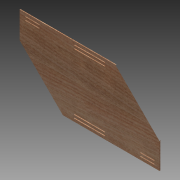
# Autodesk Inventor part: plaat
Saved by Autodesk Inventor 2015 (Build 190159000, 159)
## iProperties
Created: 2015-12-19
Part Number: plaat
Material: Generic
Document SubType Name: Modeling
Designer: david
Density: 1 g/cm^3
Appearance: Birch - Natural Polished
Author: david
Autodesk Inventor part; units mm, degrees
ref_plane "YZ Plane" through (0, 0, 0) normal (1, 0, 0) x (0, 1, 0)
ref_plane "XZ Plane" through (0, 0, 0) normal (0, 1, 0) x (-1, 0, 0)
ref_plane "XY Plane" through (0, 0, 0) normal (0, 0, 1) x (1, 0, 0)
sketch "Sketch1" plane through (0, 0, 0) normal (0, 1, 0) x (-1, 0, 0)
  line L0 (-250, 125) -> (250, 125)
  line L1 (250, 125) -> (250, -125)
  line L2 (250, -125) -> (-250, -125)
  line L3 (-250, -125) -> (-250, 125)
  line L4 (-250, 125) -> (250, -125) construction
  line L5 (250, 125) -> (-250, -125) construction
  point P0 (0, 0)
  dimension "d0" = 500
  dimension "d1" = 250
  constraints: 12 end point, 2 midpoint, 2 parallel, 1 horizontal, 1 perpendicular
  measures "d0" distance of L1.end L2.end
  measures "d1" distance of L0.end L1.end
extrude "Extrusion1" add sketch "Sketch1" along normal blind 3
sketch "Sketch3" plane through (0, 3, 0) normal (0, 1, 0) x (1, 0, 0)
  line L0 (55.5, 115.125) -> (4.5, 115.125)
  line L1 (4.5, 115.125) -> (4.5, 111.875)
  line L2 (4.5, 111.875) -> (55.5, 111.875)
  line L3 (55.5, 111.875) -> (55.5, 115.125)
  line L4 (55.5, 115.125) -> (4.5, 111.875) construction
  line L5 (4.5, 115.125) -> (55.5, 111.875) construction
  line L6 (-4.5, 115.125) -> (-55.5, 115.125)
  line L7 (-55.5, 115.125) -> (-55.5, 111.875)
  line L8 (-55.5, 111.875) -> (-4.5, 111.875)
  line L9 (-4.5, 111.875) -> (-4.5, 115.125)
  line L10 (-4.5, 115.125) -> (-55.5, 111.875) construction
  line L11 (-55.5, 115.125) -> (-4.5, 111.875) construction
  line L12 (250, 125) -> (-250, 125) projected
  line L13 (231, 115.125) -> (180, 115.125)
  line L14 (180, 115.125) -> (180, 111.875)
  line L15 (180, 111.875) -> (231, 111.875)
  line L16 (231, 111.875) -> (231, 115.125)
  line L17 (231, 115.125) -> (180, 111.875) construction
  line L18 (180, 115.125) -> (231, 111.875) construction
  line L19 (4.5, 115.125) -> (-4.5, 115.125)
  line L20 (-4.5, 115.125) -> (-4.5, 111.875)
  line L21 (-4.5, 111.875) -> (4.5, 111.875)
  line L22 (4.5, 111.875) -> (4.5, 115.125)
  line L23 (-180, 115.125) -> (-231, 115.125)
  line L24 (-231, 115.125) -> (-231, 111.875)
  line L25 (-231, 111.875) -> (-180, 111.875)
  line L26 (-180, 111.875) -> (-180, 115.125)
  line L27 (250, 125) -> (250, -125)
  line L28 (55.5, 103.625) -> (4.5, 103.625)
  line L29 (4.5, 103.625) -> (4.5, 100.375)
  line L30 (4.5, 100.375) -> (55.5, 100.375)
  line L31 (55.5, 100.375) -> (55.5, 103.625)
  line L32 (55.5, 103.625) -> (4.5, 100.375) construction
  line L33 (4.5, 103.625) -> (55.5, 100.375) construction
  line L34 (-4.5, 103.625) -> (-55.5, 103.625)
  line L35 (-55.5, 103.625) -> (-55.5, 100.375)
  line L36 (-55.5, 100.375) -> (-4.5, 100.375)
  line L37 (-4.5, 100.375) -> (-4.5, 103.625)
  line L38 (-4.5, 103.625) -> (-55.5, 100.375) construction
  line L39 (-55.5, 103.625) -> (-4.5, 100.375) construction
  line L40 (4.5, 103.625) -> (-4.5, 103.625)
  line L41 (-4.5, 103.625) -> (-4.5, 100.375)
  line L42 (-4.5, 100.375) -> (4.5, 100.375)
  line L43 (4.5, 100.375) -> (4.5, 103.625)
  line L44 (-180, 103.625) -> (-231, 103.625)
  line L45 (-231, 103.625) -> (-231, 100.375)
  line L46 (-231, 100.375) -> (-180, 100.375)
  line L47 (-180, 100.375) -> (-180, 103.625)
  line L48 (250, 113.5) -> (250, -136.5)
  line L49 (253.2147, 0) -> (-252.6779, 0)
  line L50 (231, 103.625) -> (180, 103.625)
  line L51 (180, 103.625) -> (180, 100.375)
  line L52 (180, 100.375) -> (231, 100.375)
  line L53 (231, 100.375) -> (231, 103.625)
  line L54 (231, 103.625) -> (180, 100.375) construction
  line L55 (180, 103.625) -> (231, 100.375) construction
  line L56 (55.5, -115.125) -> (4.5, -115.125)
  line L57 (4.5, -115.125) -> (4.5, -111.875)
  line L58 (4.5, -111.875) -> (55.5, -111.875)
  line L59 (55.5, -111.875) -> (55.5, -115.125)
  line L60 (55.5, -115.125) -> (4.5, -111.875) construction
  line L61 (4.5, -115.125) -> (55.5, -111.875) construction
  line L62 (-4.5, -115.125) -> (-55.5, -115.125)
  line L63 (-55.5, -115.125) -> (-55.5, -111.875)
  line L64 (-55.5, -111.875) -> (-4.5, -111.875)
  line L65 (-4.5, -111.875) -> (-4.5, -115.125)
  line L66 (-4.5, -115.125) -> (-55.5, -111.875) construction
  line L67 (-55.5, -115.125) -> (-4.5, -111.875) construction
  line L68 (250, -125) -> (-250, -125)
  line L69 (231, -115.125) -> (180, -115.125)
  line L70 (180, -115.125) -> (180, -111.875)
  line L71 (180, -111.875) -> (231, -111.875)
  line L72 (231, -111.875) -> (231, -115.125)
  line L73 (231, -115.125) -> (180, -111.875) construction
  line L74 (180, -115.125) -> (231, -111.875) construction
  line L75 (4.5, -115.125) -> (-4.5, -115.125)
  line L76 (-4.5, -115.125) -> (-4.5, -111.875)
  line L77 (-4.5, -111.875) -> (4.5, -111.875)
  line L78 (4.5, -111.875) -> (4.5, -115.125)
  line L79 (-180, -115.125) -> (-231, -115.125)
  line L80 (-231, -115.125) -> (-231, -111.875)
  line L81 (-231, -111.875) -> (-180, -111.875)
  line L82 (-180, -111.875) -> (-180, -115.125)
  line L83 (4.5, -103.625) -> (-4.5, -103.625)
  line L84 (-4.5, -100.375) -> (4.5, -100.375)
  line L85 (-4.5, -100.375) -> (-4.5, -103.625)
  line L86 (-4.5, -103.625) -> (-4.5, -100.375)
  line L87 (-55.5, -100.375) -> (-4.5, -100.375)
  line L88 (-55.5, -103.625) -> (-55.5, -100.375)
  line L89 (-4.5, -103.625) -> (-55.5, -100.375) construction
  line L90 (-55.5, -103.625) -> (-4.5, -100.375) construction
  line L91 (-4.5, -103.625) -> (-55.5, -103.625)
  line L92 (4.5, -103.625) -> (4.5, -100.375)
  line L93 (4.5, -100.375) -> (4.5, -103.625)
  line L94 (55.5, -103.625) -> (4.5, -103.625)
  line L95 (4.5, -100.375) -> (55.5, -100.375)
  line L96 (55.5, -103.625) -> (4.5, -100.375) construction
  line L97 (4.5, -103.625) -> (55.5, -100.375) construction
  line L98 (55.5, -100.375) -> (55.5, -103.625)
  line L99 (-180, -100.375) -> (-180, -103.625)
  line L100 (-180, -103.625) -> (-231, -103.625)
  line L101 (-231, -100.375) -> (-180, -100.375)
  line L102 (-231, -103.625) -> (-231, -100.375)
  line L103 (180, -103.625) -> (180, -100.375)
  line L104 (231, -103.625) -> (180, -103.625)
  line L105 (180, -100.375) -> (231, -100.375)
  line L106 (231, -103.625) -> (180, -100.375) construction
  line L107 (180, -103.625) -> (231, -100.375) construction
  line L108 (231, -100.375) -> (231, -103.625)
  point P0 (0, 0)
  point P1 (30, 113.5)
  point P2 (-30, 113.5)
  point P3 (205.5, 113.5)
  point P4 (0, -11.5)
  point P5 (30, 102)
  point P6 (-30, 102)
  point P7 (-250, 113.5)
  point P8 (205.5, 102)
  point P9 (30, -113.5)
  point P10 (-30, -113.5)
  point P11 (205.5, -113.5)
  point P12 (250, -113.5)
  point P13 (-250, -113.5)
  point P14 (-30, -102)
  point P15 (30, -102)
  point P16 (205.5, -102)
  dimension "d28" = 51
  dimension "d29" = 3.25
  dimension "d30" = 51
  dimension "d31" = 3.25
  dimension "d32" = 4.5
  dimension "d33" = 9
  dimension "d34" = 9.875
  dimension "d35" = 9.875
  dimension "d36" = 51
  dimension "d37" = 3.25
  dimension "d38" = 124.5
  dimension "d39" = 9.875
  dimension "d40" = 51
  dimension "d41" = 3.25
  dimension "d42" = 124.5
  dimension "d43" = 9.875
  dimension "d46" = 11.5
  dimension "d53" = 11.5
  constraints: 216 end point, 45 symmetric about line, 24 midpoint, 10 parallel, 6 horizontal, 5 perpendicular, 3 vertical, 1 collinear, 51 other
  measures "d28" distance of L2.end L1.end
  measures "d29" distance of L1.end L0.end
  measures "d30" distance of L8.end L7.end
  measures "d31" distance of L7.end L6.end
  measures "d32" distance from line of L9 point (0, 0)
  measures "d33" distance between parallel lines of L1 L9
  measures "d34" distance between parallel lines of L12 L6
  measures "d35" distance between parallel lines of L12 L0
  measures "d36" distance of L15.end L14.end
  measures "d37" distance of L14.end L13.end
  measures "d38" distance of L0.start L13.end
  measures "d39" distance between parallel lines of L12 L13
  measures "d40" distance of L25.end L24.end
  measures "d41" distance of L24.end L23.end
  measures "d42" horizontal distance of L7.end L23.start
  measures "d43" distance between parallel lines of L12 L23
  measures "d46" distance of point (0, 0) point (0, -11.5)
  measures "d53" distance of L14.end L51.end
extrude "Extrusion3" cut sketch "Sketch3" against normal blind 10
body "Solid1"
